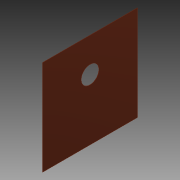
# Autodesk Inventor part: 2221A_Copper Box Side_Hole_V1
Saved by Autodesk Inventor 2020 (Build 240168000, 168)
## iProperties
Created: 2017-08-01
Part Number: 2221A_Copper Box Side_Hole_V1
Material: Copper
Document SubType Name: Modeling
Designer: MPI
Density: 8.94 g/cm^3
Appearance: Copper - Satin
Author: MPI
Autodesk Inventor part; units mm, degrees
ref_plane "YZ Plane" through (0, 0, 0) normal (1, 0, 0) x (0, 1, 0)
ref_plane "XZ Plane" through (0, 0, 0) normal (0, 1, 0) x (-1, 0, 0)
ref_plane "XY Plane" through (0, 0, 0) normal (0, 0, 1) x (1, 0, 0)
sketch "Sketch1" plane through (0, 0, 0) normal (1, 0, 0) x (0, 1, 0)
  line L0 (-304.8, 304.8) -> (304.8, 304.8)
  line L1 (304.8, 304.8) -> (304.8, -304.8)
  line L2 (304.8, -304.8) -> (-304.8, -304.8)
  line L3 (-304.8, -304.8) -> (-304.8, 304.8)
  line L4 (-304.8, 304.8) -> (304.8, -304.8) construction
  line L5 (304.8, 304.8) -> (-304.8, -304.8) construction
  point P0 (0, 0)
  dimension "d0" = 609.6
  dimension "d1" = 609.6
  constraints: 12 end point, 2 midpoint, 2 parallel, 1 horizontal, 1 perpendicular
  measures "d0" distance of L1.end L2.end
  measures "d1" distance of L0.end L1.end
extrude "Extrusion1" add sketch "Sketch1" along normal blind 1.0668
sketch "Sketch2" plane through (1.0668, 0, 0) normal (1, 0, 0) x (0, 0, -1)
  circle A0 centre (0, 85.725) radius 57.15
  line L0 (-304.8, -304.8) -> (304.8, -304.8) projected
  dimension "d4" = 114.3
  dimension "d7" = 390.525
  constraints: 1 centre point, 1 coincident
  measures "d4" diameter of A0
  measures "d7" distance from line of L0 point (0, 85.725)
extrude "Extrusion2" cut sketch "Sketch2" against normal through all
body "Solid1"
